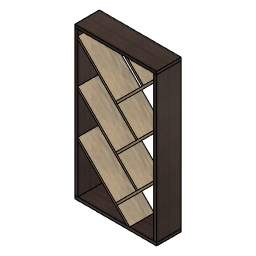
Modern Book Shelf (Autodesk Fusion 360 design; units mm, degrees)
Autodesk Fusion 360 part; units mm, degrees
sketch "Sketch1" plane through (0, 0, 0) normal (0, 1, 0) x (1, 0, 0)
  line L0 (0, 0) -> (1000, 0)
  line L1 (1000, 0) -> (1000, -1850)
  line L2 (1000, -1850) -> (0, -1850)
  line L3 (0, -1850) -> (0, 0)
  dimension "d4" = 1000
  dimension "d5" = 1850
  constraint horizontal L0
  constraint vertical L1
  constraint horizontal L2
  constraint vertical L3
  constraint coincident L0.start L3.end
  measures "d4" distance of L0.start L0.end
  measures "d5" distance of L0.start L2.end
extrude "Extrude1" add sketch "Sketch1" along normal blind 300 makes body 1
extrude "Extrude1'" add 1 faces at (0, 100, 1233.3333) along direction (1, 0, 0) blind 36 separate body on bodies 1 makes body 2 in component "Left"
extrude "Extrude1''" add 1 faces at (333.3333, 100, 0) along direction (0, 0, 1) blind 36 separate body on bodies 1 makes body 3 in component "Bottom"
extrude "Extrude1'''" add 1 faces at (1000, 100, 616.6667) along direction (-1, 0, 0) blind 36 separate body on bodies 1 makes body 4 in component "Right"
extrude "Extrude1''''" add 1 faces at (666.6667, 100, 1850) along direction (0, 0, -1) blind 36 separate body on bodies 1 makes body 5 in component "Top"
combine "Combine1" operation cut target body 2 tool bodies 5 3 keep tools in component "Left"
combine "Combine1'" operation cut target body 4 tool bodies 5 3 keep tools in component "Right"
sketch "Bottom Shelves" plane through (0, 0, 0) normal (0, 1, 0) x (1, 0, 0) in component "Shelves"
  line L0 (36, -671) -> (671, -36)
  line L1 (0, -36) -> (1000, -36)
  line L2 (36, -1814) -> (36, -36)
  line L3 (36, -635.6447) -> (635.6447, -36)
  line L4 (964, -635.6447) -> (517.6777, -189.3223)
  line L5 (964, -36) -> (964, -1814)
  line L6 (964, -671) -> (500, -207)
  dimension "d18" = 635
  dimension "d19" = 135
  dimension "d20" = 25
  dimension "d23" = 25
  constraint coincident L0.start L2
  constraint coincident L0.end L1
  constraint parallel L0 L3
  constraint coincident L2 L3.start
  constraint coincident L1 L3.end
  constraint coincident L0 L4.end
  constraint coincident L4.start L5
  constraint perpendicular L0 L4
  constraint coincident L5 L6.start
  constraint coincident L0 L6.end
  constraint perpendicular L0 L6
  constraint horizontal L0.start L6.start
  measures "d18" distance of L0.start L1
  measures "d19" angle of L0 L1
  measures "d20" distance of L0 L3
  measures "d23" distance of L4 L6
extrude "Extrude1'''''" add sketch "Bottom Shelves" along normal up to surface (300 mm away) separate body contours L0 L1 L2 L3 makes body 6 in component "Shelves"
extrude "Extrude2" add sketch "Bottom Shelves" along normal up to surface (300 mm away) separate body contours L0 L4 L5 L6 makes body 7 in component "Shelves"
copy_body "Body->Comp1" bodies 6 removing the originals makes body 8 in component "Shelf"
copy_body "Body->Comp2" bodies 7 removing the originals makes body 9 in component "Pillar"
sketch "Sketch2" plane through (0, 0, 0) normal (0, -1, 0) x (1, 0, 0) in component "Shelves"
  line L0 (0, 0) -> (1000, 0)
  line L1 (1000, 0) -> (1000, 36)
  line L2 (1000, 36) -> (0, 36)
  line L3 (0, 36) -> (0, 0)
  line L4 (36, 1814) -> (36, 36)
  line L5 (36, 1208) -> (768.5, 475.5)
  line L6 (964, 671) -> (500, 207)
  line L7 (36, 1172.6447) -> (750.8223, 457.8223)
  point P0 (36, 1208)
  point P1 (36, 671)
  point P2 (36, 1745)
  dimension "d26" = 537
  dimension "d27" = 537
  dimension "d28" = 25
  constraint coincident P0 L4
  constraint coincident L4 P2
  constraint coincident P0 L5.start
  constraint coincident L5.end L6
  constraint perpendicular L5 L6
  constraint coincident L4 L7.start
  constraint coincident L6 L7.end
  constraint parallel L5 L7
  measures "d26" distance of P0 P1
  measures "d27" distance of P0 P2
  measures "d28" distance of L5 L7
extrude "Extrude3" add sketch "Sketch2" against normal up to surface (300 mm away) separate body contours L4 L5 L6 L7 makes body 10 in component "Shelves"
copy_body "Body->Comp3" bodies 10 removing the originals makes body 11 in component "Shelf2"
pattern_linear "00000000-0000-0000-0000-000000000000" [suppressed] in component "Shelves"
pattern_linear "00000000-0000-0000-0000-000000000000'" [suppressed] in component "Shelves"
sketch "Sketch3" plane through (0, 0, 0) normal (0, -1, 0) x (1, 0, 0) in component "Shelves"
  line L0 (1000, 1850) -> (0, 1850)
  line L1 (0, 1850) -> (0, 1814)
  line L2 (0, 1814) -> (1000, 1814)
  line L3 (1000, 1814) -> (1000, 1850)
  line L4 (644, 1814) -> (838.5, 1619.5)
  line L5 (964, 1745) -> (500, 1281)
  line L6 (608.6447, 1814) -> (820.8223, 1601.8223)
  point P0 (964, 1814)
  dimension "d39" = 320
  dimension "d40" = 25
  constraint coincident L2 L4.start
  constraint coincident L4.end L5
  constraint perpendicular L4 L5
  constraint coincident L2 L6.start
  constraint coincident L5 L6.end
  constraint parallel L4 L6
  measures "d39" distance of L4.start P0
  measures "d40" distance of L4 L6
extrude "Extrude4" add sketch "Sketch3" against normal up to surface (300 mm away) separate body contours L2 L4 L5 L6 makes body 12 in component "Shelves"
copy_body "Body->Comp4" bodies 12 removing the originals makes body 13 in component "Small Pillar"
component "Left" placed x (1, 0, 0) y (0, 1, 0) z (0, 0, 1) at (0, 0, 0)
component "Bottom" placed x (1, 0, 0) y (0, 1, 0) z (0, 0, 1) at (0, 0, 0)
component "Right" placed x (1, 0, 0) y (0, 1, 0) z (0, 0, 1) at (0, 0, 0)
component "Top" placed x (1, 0, 0) y (0, 1, 0) z (0, 0, 1) at (0, 0, 0)
component "Shelves" placed x (1, 0, 0) y (0, 1, 0) z (0, 0, 1) at (0, 0, 0)
component "Shelf" placed x (1, 0, 0) y (0, 1, 0) z (0, 0, 1) at (0, 0, 0) in component "Shelves"
component "Pillar" placed x (1, 0, 0) y (0, 1, 0) z (0, 0, 1) at (0, 0, 0) in component "Shelves"
component "Shelf2" placed x (1, 0, 0) y (0, 1, 0) z (0, 0, 1) at (0, 0, 0) in component "Shelves"
component "Shelf2" placed x (1, 0, 0) y (0, 1, 0) z (0, 0, 1) at (0, 0, 537) in component "Shelves"
component "Pillar" placed x (1, 0, 0) y (0, 1, 0) z (0, 0, 1) at (0, 0, 537) in component "Shelves"
component "Pillar" placed x (1, 0, 0) y (0, 1, 0) z (0, 0, 1) at (0, 0, 1074) in component "Shelves"
component "Small Pillar" placed x (1, 0, 0) y (0, 1, 0) z (0, 0, 1) at (0, 0, 0) in component "Shelves"
hidden bodies 1
equation "Height = 1850 mm"
equation "Width = 1000 mm"
equation "Depth = 300 mm"
equation "d4 = Width"
equation "d5 = Height"
equation "d6 = Depth"
equation "BoardT1 = 36 mm"
equation "BoardT2 = 25 mm"
equation "d10 = -( 36.00 mm )"
equation "d12 = -( 36.00 mm )"
equation "d14 = -( 36.00 mm )"
equation "d16 = -( 36.00 mm )"
equation "d19 = 180 deg - 45 deg"
equation "d20 = BoardT2"
equation "d23 = BoardT2"
equation "d27 = d26"
equation "d28 = BoardT2"
equation "d40 = BoardT2"
named bodies: "Shelf", "Pillar", "Shelf2", "Small Pillar"
